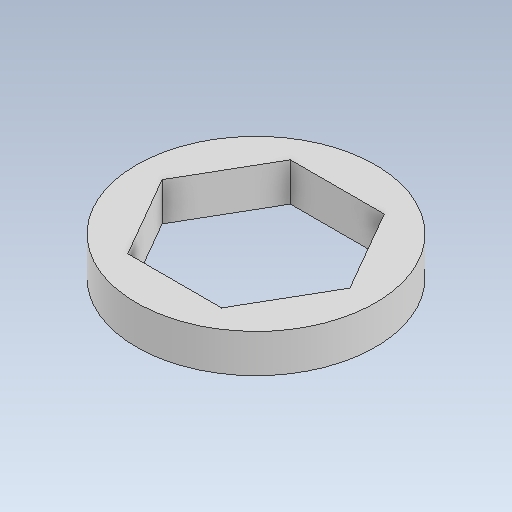
# Autodesk Inventor part: 3mmHEXSPACER
Saved by Autodesk Inventor 2020 (Build 240168000, 168)
## iProperties
Created: 2021-01-14
Part Number: 3mmHEXSPACER
Material: Generic
Document SubType Name: Modeling
Designer: lucky
Density: 1 g/cm^3
Appearance: Default
Mass: 0.403216 g
Surface Area: 5.773 cm^2
Volume: 0.403216 cm^3
Author: lucky
Autodesk Inventor part; units mm, degrees
ref_plane "YZ Plane" through (0, 0, 0) normal (1, 0, 0) x (0, 1, 0)
ref_plane "XZ Plane" through (0, 0, 0) normal (0, 1, 0) x (-1, 0, 0)
ref_plane "XY Plane" through (0, 0, 0) normal (0, 0, 1) x (1, 0, 0)
sketch "Sketch1" plane through (0, 0, 0) normal (0, 1, 0) x (-1, 0, 0)
  line L0 (-6.35, -3.6662) -> (-6.35, 3.6662)
  line L1 (-6.35, 3.6662) -> (0, 7.3323)
  line L2 (0, 7.3323) -> (6.35, 3.6662)
  line L3 (6.35, 3.6662) -> (6.35, -3.6662)
  line L4 (6.35, -3.6662) -> (0, -7.3323)
  line L5 (0, -7.3323) -> (-6.35, -3.6662)
  circle A0 centre (0, 0) radius 6.35
  circle A1 centre (0, 0) radius 9.35
  dimension "d0" = 12.7
  dimension "d1" = 3
  constraints: 12 end point, 2 centre point, 2 coincident, 1 tangent, 1 vertical alignment, 13 other
  measures "d0" distance between parallel lines of L0 L3
  measures "d1" radial gap between concentric circles of A0 A1
extrude "Extrusion1" add sketch "Sketch1" along normal blind 3 contours L0 A0 L5 | L0 L1 A0 | A0 | A0 L4 L5 | L1 L2 A0 | A0 L3 L4 | L2 L3 A0 | A1
sketch "Sketch2" plane through (0, 3, 0) normal (0, 1, 0) x (1, 0, 0)
  line L0 (-7.347, 0) -> (-3.6735, 6.3627)
  line L1 (-3.6735, 6.3627) -> (3.6735, 6.3627)
  line L2 (3.6735, 6.3627) -> (7.347, 0)
  line L3 (7.347, 0) -> (3.6735, -6.3627)
  line L4 (3.6735, -6.3627) -> (-3.6735, -6.3627)
  line L5 (-3.6735, -6.3627) -> (-7.347, 0)
  point P0 (0, 0)
  point P1 (0, 0)
  dimension "d4" = 12.7254
  constraints: 12 end point, 1 coincident, 1 horizontal alignment, 13 other
  measures "d4" distance between parallel lines of L0 L3
extrude "Extrusion2" cut sketch "Sketch2" against normal blind 3
body "Solid1"
